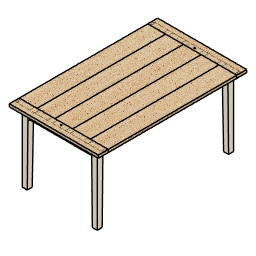
Farmhouse Table 2021 (Autodesk Fusion 360 design; units mm, degrees)
Autodesk Fusion 360 part; units mm, degrees
note: some values were not read from the file. Chosen so that the rebuilt part matches the saved one: which face or edge a step refers to; where a step ends. Set by a fixed rule: which sketch regions a step uses.
sketch "Sketch1" plane through (0, 0, 0) normal (1, 0, 0) x (0, 0, -1) in component "Breadboard"
  line L0 (0, 0) -> (-101.6, 0)
  line L1 (-101.6, 0) -> (-101.6, 28.575)
  line L2 (-101.6, 28.575) -> (0, 28.575)
  line L3 (0, 28.575) -> (0, 0)
  dimension "d1" = 28.575
  dimension "d2" = 101.6
  dimension "d215" = 0
  dimension "d216" = 0
  dimension "d217" = 0
  dimension "d218" = 0
  dimension "d275" = 0
  dimension "d276" = 0
  dimension "d277" = 0
  dimension "d278" = 0
  constraint horizontal L0
  constraint vertical L1
  constraint horizontal L2
  constraint vertical L3
  constraint coincident L0.start L3.end
  measures "d1" distance of L0.start L2.end
  measures "d2" distance of L0.start L0.end
extrude "Extrude1" add sketch "Sketch1" along normal blind 914.4 makes body 1 in component "Breadboard"
sketch "Sketch2" plane through (0, 0, 0) normal (0, 0, -1) x (-1, 0, 0) in component "Breadboard"
  line L0 (0, 0) -> (0, 28.575)
  line L1 (0, 28.575) -> (-914.4, 28.575)
  line L2 (-914.4, 28.575) -> (-914.4, 0)
  line L3 (-914.4, 0) -> (0, 0)
  line L4 (-901.7, 7.9375) -> (-12.7, 7.9375)
  line L5 (-12.7, 7.9375) -> (-12.7, 20.6375)
  line L6 (-12.7, 20.6375) -> (-901.7, 20.6375)
  line L7 (-901.7, 20.6375) -> (-901.7, 7.9375)
  line L8 (-901.7, 20.6375) -> (-901.7, 28.575) construction
  line L9 (-901.7, 7.9375) -> (-901.7, 0) construction
  line L10 (-12.7, 20.6375) -> (0, 20.6375) construction
  line L11 (-901.7, 20.6375) -> (-914.4, 20.6375) construction
  dimension "d7" = 12.7
  dimension "d11" = 12.7
  constraint horizontal L4
  constraint vertical L5
  constraint horizontal L6
  constraint vertical L7
  constraint coincident L1 L8.end
  constraint perpendicular L1 L8
  constraint coincident L3 L9.end
  constraint vertical L9
  constraint equal L8 L9
  constraint coincident L0 L10.end
  constraint coincident L2 L11.end
  constraint horizontal L11
  constraint horizontal L10
  constraint equal L10 L11
  measures "d7" vertical distance of L4.start L6.end
  measures "d11" distance of L2 L7
extrude "Extrude2" cut sketch "Sketch2" against normal blind 50.8 contours L4 L5 L6 L7 bodies 1 in component "Breadboard"
sketch "Sketch3" plane through (0, 28.575, 0) normal (0, 1, 0) x (-1, 0, 0) in component "Breadboard"
  line L0 (0, 0) -> (0, 101.6)
  line L1 (0, 101.6) -> (-914.4, 101.6)
  line L2 (-914.4, 101.6) -> (-914.4, 0)
  line L3 (-914.4, 0) -> (0, 0)
  line L4 (-457.2, 0) -> (-457.2, 25.4) construction
  circle A0 centre (-457.2, 25.4) radius 6.35
  dimension "d15" = 25.4
  dimension "d17" = 12.7
  constraint coincident L3 L4.start
  constraint perpendicular L3 L4
  constraint midpoint L3 L4.start
  constraint coincident L4.end A0.centre
  measures "d15" vertical distance of L4.start L4.end
  measures "d17" diameter of A0
extrude "Extrude3" cut sketch "Sketch3" against normal through all contours A0 bodies 1 in component "Breadboard"
sketch "Sketch1 (2)" plane through (0, 0, 0) normal (0, 0, 1) x (1, 0, 0) in component "Board"
  line L0 (0, 0) -> (182.88, 0)
  line L1 (182.88, 0) -> (182.88, 28.575)
  line L2 (182.88, 28.575) -> (0, 28.575)
  line L3 (0, 28.575) -> (0, 0)
  line L4 (0, 28.575) -> (914.4, 28.575)
  dimension "d22" = 182.88
  constraint horizontal L0
  constraint vertical L1
  constraint horizontal L2
  constraint vertical L3
  constraint coincident L1.end L4
  constraint coincident L0.start L3.end
  measures "d22" horizontal distance of L0.start L0.end
extrude "Extrude1'" add sketch "Sketch1 (2)" against normal blind 1320.8 separate body makes body 2 in component "Board"
ref_plane "WorkPlane1" through (91.44, 14.2875, -660.4) normal (0, 0, 1) x (1, 0, 0) in component "Board"
sketch "Sketch2 (2)" plane through (0, 0, 0) normal (0, 0, 1) x (1, 0, 0) in component "Board"
  line L0 (0, 0) -> (182.88, 0)
  line L1 (182.88, 0) -> (182.88, 28.575)
  line L2 (182.88, 28.575) -> (0, 28.575)
  line L3 (0, 28.575) -> (0, 0)
  line L4 (25.4, 7.9375) -> (157.48, 7.9375)
  line L5 (157.48, 7.9375) -> (157.48, 20.6375)
  line L6 (157.48, 20.6375) -> (25.4, 20.6375)
  line L7 (25.4, 20.6375) -> (25.4, 7.9375)
  line L8 (157.48, 7.9375) -> (157.48, 0) construction
  line L9 (157.48, 20.6375) -> (157.48, 28.575) construction
  line L10 (91.44, 28.575) -> (91.44, 0) construction
  dimension "d25" = 12.7
  dimension "d26" = 25.4
  constraint horizontal L4
  constraint vertical L5
  constraint horizontal L6
  constraint vertical L7
  constraint coincident L0 L8.end
  constraint coincident L2 L9.end
  constraint equal L8 L9
  constraint vertical L8
  constraint vertical L9
  constraint midpoint L2 L10.start
  constraint midpoint L0 L10.end
  constraint symmetric L5 L7 L10
  measures "d25" vertical distance of L4.start L6.end
  measures "d26" distance of L3 L7
extrude "Extrude2'" add sketch "Sketch2 (2)" along normal blind 50.8 contours L4 L5 L6 L7 bodies 2 in component "Board"
mirror "Mirror1" about plane through (91.44, 14.2875, -660.4) normal (0, 0, 1) of "Extrude2'" in component "Board"
sketch "Sketch1 (3)" plane through (0, 0, 0) normal (0, 0, 1) x (1, 0, 0) in component "Centerboard"
  line L0 (0, 0) -> (182.88, 0)
  line L1 (182.88, 0) -> (182.88, 28.575)
  line L2 (182.88, 28.575) -> (0, 28.575)
  line L3 (0, 28.575) -> (0, 0)
  line L4 (0, 28.575) -> (914.4, 28.575)
  dimension "d22_1" = 182.88
  constraint horizontal L0
  constraint vertical L1
  constraint horizontal L2
  constraint vertical L3
  constraint coincident L1.end L4
  constraint coincident L0.start L3.end
  measures "d22_1" horizontal distance of L0.start L0.end
extrude "Extrude1''" add sketch "Sketch1 (3)" against normal blind 1320.8 separate body makes body 3 in component "Centerboard"
ref_plane "WorkPlane1" through (91.44, 14.2875, -660.4) normal (0, 0, 1) x (1, 0, 0) in component "Centerboard"
sketch "Sketch2 (3)" plane through (0, 0, 0) normal (0, 0, 1) x (1, 0, 0) in component "Centerboard"
  line L0 (0, 0) -> (182.88, 0)
  line L1 (182.88, 0) -> (182.88, 28.575)
  line L2 (182.88, 28.575) -> (0, 28.575)
  line L3 (0, 28.575) -> (0, 0)
  line L4 (25.4, 7.9375) -> (157.48, 7.9375)
  line L5 (157.48, 7.9375) -> (157.48, 20.6375)
  line L6 (157.48, 20.6375) -> (25.4, 20.6375)
  line L7 (25.4, 20.6375) -> (25.4, 7.9375)
  line L8 (157.48, 7.9375) -> (157.48, 0) construction
  line L9 (157.48, 20.6375) -> (157.48, 28.575) construction
  line L10 (25.4, 20.6375) -> (25.4, 7.9375)
  line L11 (91.44, 28.575) -> (91.44, 0)
  dimension "d25_1" = 12.7
  dimension "d26_1" = 25.4
  constraint horizontal L4
  constraint vertical L5
  constraint horizontal L6
  constraint vertical L7
  constraint coincident L0 L8.end
  constraint coincident L2 L9.end
  constraint equal L8 L9
  constraint vertical L8
  constraint vertical L9
  measures "d25_1" vertical distance of L4.start L6.end
  measures "d26_1" distance of L3 L7
extrude "Extrude2''" add sketch "Sketch2 (3)" along normal blind 50.8 contours L4 L5 L6 L11 | L4 L6 L7 L10 L11 bodies 3 in component "Centerboard"
mirror "Mirror1'" about plane through (91.44, 14.2875, -660.4) normal (0, 0, 1) of "Extrude2''" in component "Centerboard"
sketch "Sketch3 (2)" plane through (0, 0, 0) normal (0, 1, 0) x (1, 0, 0) in component "Centerboard"
  circle A0 centre (91.44, -25.4) radius 6.35
  line L0 (25.4, -50.8) -> (157.48, -50.8)
  line L1 (91.44, -25.4) -> (91.44, -50.8) construction
  dimension "d30" = 12.7
  dimension "d31" = 25.4
  constraint coincident A0.centre L1.start
  constraint midpoint L0 L1.end
  constraint vertical L1
  measures "d30" diameter of A0
  measures "d31" vertical distance of A0.centre L1.end
extrude "Extrude3'" cut sketch "Sketch3 (2)" along normal up to surface (20.6375 mm away) bodies 3 in component "Centerboard"
mirror "Mirror2" about plane through (91.44, 14.2875, -660.4) normal (0, 0, 1) of "Extrude3'" in component "Centerboard"
sketch "Sketch1 (4)" plane through (0, 0, 0) normal (0, 1, 0) x (1, 0, 0) in component "Dowel"
  circle A0 centre (457.2, -25.4) radius 6.35
  circle A1 centre (457.2, -25.4) radius 6.35
  point P0 (463.55, -25.4)
  constraint coincident A0 P0
  constraint concentric A0 A1
extrude "Extrude1'''" add sketch "Sketch1 (4)" along normal blind 28.575 separate body makes body 4 in component "Dowel"
sketch "Sketch1 (5)" plane through (0, 0, 0) normal (0, 1, 0) x (1, 0, 0) in component "leg"
  line L0 (73.025, -28.575) -> (130.175, -28.575)
  line L1 (130.175, -28.575) -> (130.175, 28.575)
  line L2 (130.175, 28.575) -> (73.025, 28.575)
  line L3 (73.025, 28.575) -> (73.025, -28.575)
  line L4 (0, 0) -> (914.4, 0)
  line L5 (0, -101.6) -> (0, 0)
  line L6 (73.025, -28.575) -> (0, -28.575) construction
  line L7 (0, -101.6) -> (914.4, -101.6)
  line L8 (73.025, -28.575) -> (73.025, -101.6) construction
  dimension "d45" = 57.15
  dimension "d46" = 28.575
  constraint horizontal L0
  constraint vertical L1
  constraint horizontal L2
  constraint vertical L3
  constraint equal L0 L3
  constraint coincident L5 L6.end
  constraint coincident L7 L8.end
  constraint perpendicular L0 L8
  constraint horizontal L6
  constraint equal L6 L8
  measures "d45" horizontal distance of L0.start L0.end
  measures "d46" distance of L0 L4
extrude "Extrude1''''" add sketch "Sketch1 (5)" against normal blind 708.025 separate body makes body 5 in component "leg"
ref_plane "WorkPlane1" through (130.175, 0, -28.575) normal (0.707107, 0, 0.707107) x (0, 1, 0) in component "leg"
sketch "Sketch2 (4)" plane through (130.175, 0, 0) normal (1, 0, 0) x (0, 0, -1) in component "leg"
  line L0 (28.575, 0) -> (-28.575, 0)
  line L1 (-28.575, 0) -> (-28.575, -708.025)
  line L2 (-28.575, -708.025) -> (28.575, -708.025)
  line L3 (28.575, -708.025) -> (28.575, 0)
  line L4 (28.575, -89.154) -> (22.225, -708.025)
  dimension "d51" = 618.871
  dimension "d52" = 50.8
  constraint coincident L3 L4.start
  constraint coincident L2 L4.end
  measures "d51" distance of L2 L4.start
  measures "d52" distance of L1 L4.end
extrude "Extrude2'''" cut sketch "Sketch2 (4)" against normal up to surface (57.15 mm away) contours L2 L3 L4 bodies 5 in component "leg"
mirror "Mirror1''" about plane through (130.175, 0, -28.575) normal (0.707107, 0, 0.707107) of "Extrude2'''" in component "leg"
sketch "Sketch3 (3)" plane through (130.175, 0, 0) normal (1, 0, 0) x (0, 0, -1) in component "leg"
  line L0 (-28.575, -89.154) -> (28.575, -89.154)
  line L1 (28.575, -89.154) -> (28.575, 0)
  line L2 (28.575, 0) -> (-28.575, 0)
  line L3 (-28.575, 0) -> (-28.575, -89.154)
  line L4 (-6.35, 0) -> (6.35, 0)
  line L5 (6.35, 0) -> (6.35, -88.9)
  line L6 (6.35, -88.9) -> (-6.35, -88.9)
  line L7 (-6.35, -88.9) -> (-6.35, 0)
  dimension "d58" = 12.7
  dimension "d59" = 88.9
  constraint horizontal L4
  constraint vertical L5
  constraint horizontal L6
  constraint vertical L7
  constraint coincident L2 L4.start
  constraint midpoint L2 L4
  measures "d58" horizontal distance of L5.end L6.end
  measures "d59" vertical distance of L4.end L5.end
extrude "Extrude3''" cut sketch "Sketch3 (3)" against normal blind 25.4 contours L2 L4 L5 L6 L7 bodies 5 in component "leg"
mirror "Mirror2'" about plane through (130.175, 0, -28.575) normal (0.707107, 0, 0.707107) of "Extrude3''" in component "leg"
ref_plane "WorkPlane1" through (457.2, 14.2875, 50.8) normal (1, 0, 0) x (0, 0, -1)
ref_plane "WorkPlane2" through (457.2, 14.2875, -507.9861) normal (0, 0, 1) x (0, -1, 0)
mirror "MirrorComponent1" about plane through (0, 0, 0) normal (0, 0, 1) of bodies 5 makes body 6 in component "leg (1)"
mirror "MirrorComponent2" about plane through (0, 0, 0) normal (0, 0, 1) of bodies 5 makes body 7 in component "leg (2)"
mirror "MirrorComponent2'" about plane through (0, 0, 0) normal (0, 0, 1) of bodies 6 makes body 8 in component "leg (3)"
sketch "Sketch1 (6)" plane through (130.175, 0, 0) normal (1, 0, 0) x (0, 0, -1) in component "EndRail"
  line L0 (-6.35, -88.9) -> (-6.35, 0)
  line L1 (-6.35, 0) -> (-28.575, 0)
  line L2 (-28.575, 0) -> (-28.575, -89.154)
  line L3 (-28.575, -89.154) -> (28.575, -89.154)
  line L4 (28.575, -89.154) -> (28.575, 0)
  line L5 (28.575, 0) -> (6.35, 0)
  line L6 (6.35, 0) -> (6.35, -88.9)
  line L7 (-11.1125, 0) -> (11.1125, 0)
  line L8 (11.1125, 0) -> (11.1125, -88.9)
  line L9 (11.1125, -88.9) -> (-11.1125, -88.9)
  line L10 (-11.1125, -88.9) -> (-11.1125, 0)
  line L11 (6.35, -88.9) -> (-6.35, -88.9)
  line L12 (6.35, -88.9) -> (-6.35, -88.9)
  dimension "d63" = 22.225
  dimension "d211" = 0
  dimension "d212" = 0
  dimension "d213" = 0
  dimension "d214" = 0
  dimension "d271" = 0
  dimension "d272" = 0
  dimension "d273" = 0
  dimension "d274" = 0
  constraint horizontal L7
  constraint vertical L8
  constraint horizontal L9
  constraint vertical L10
  constraint midpoint L9 L11
  constraint collinear L1 L7
  measures "d63" horizontal distance of L8.end L9.end
extrude "Extrude1'''''" add sketch "Sketch1 (6)" along normal up to near side of body 6 placed x (-1, 0, 0) y (0, 1, 0) z (0, 0, -1) at (914.4, 0, 0) separate body contours L0 L1 L7 L9 L10 | L0 L6 L7 L9 L11 L12 | L5 L6 L7 L8 L9 makes body 9 in component "EndRail"
sketch "Sketch2 (5)" plane through (104.775, 0, 0) normal (1, 0, 0) x (0, 0, -1) in component "EndRail"
  line L0 (-6.35, -88.9) -> (3.175, -88.9)
  line L1 (3.175, 0) -> (-6.35, 0)
  line L2 (-6.35, 0) -> (-6.35, -88.9)
  line L3 (-6.35, 0) -> (3.175, 0)
  line L4 (3.175, 0) -> (3.175, -88.9)
  line L5 (3.175, -88.9) -> (-6.35, -88.9)
  line L6 (-6.35, -88.9) -> (-6.35, 0)
  line L7 (3.175, -88.9) -> (3.175, 0)
  constraint horizontal L3
  constraint vertical L4
  constraint horizontal L5
  constraint vertical L6
  constraint coincident L0.end L4.end
  constraint coincident L1.end L2.start
extrude "Extrude2''''" add sketch "Sketch2 (5)" along normal up to surface (25.4 mm away) bodies 9 in component "EndRail"
mirror "Mirror1'''" about plane through (457.2, 14.2875, 50.8) normal (1, 0, 0) of "Extrude2''''" in component "EndRail"
mirror "MirrorComponent3" about plane through (0, 0, 0) normal (0, 0, 1) of bodies 9 makes body 10 in component "EndRail (1)"
sketch "Sketch1 (7)" plane through (0, 0, -28.575) normal (0, 0, -1) x (-1, 0, 0) in component "SideRail"
  line L0 (-95.25, 0) -> (-95.25, -88.9)
  line L1 (-107.95, -88.9) -> (-107.95, 0)
  line L2 (-107.95, 0) -> (-130.175, 0)
  line L3 (-130.175, 0) -> (-130.175, -89.154)
  line L4 (-130.175, -89.154) -> (-73.025, -89.154)
  line L5 (-73.025, -89.154) -> (-73.025, 0)
  line L6 (-73.025, 0) -> (-95.25, 0)
  line L7 (-95.25, -88.9) -> (-107.95, -88.9)
sketch "Sketch2 (6)" plane through (0, 0, -28.575) normal (0, 0, -1) x (1, 0, 0) in component "SideRail"
  line L0 (112.7125, 0) -> (90.4875, 0)
  line L1 (90.4875, 0) -> (90.4875, 88.9)
  line L2 (90.4875, 88.9) -> (112.7125, 88.9)
  line L3 (112.7125, 88.9) -> (112.7125, 0)
  line L4 (107.95, 88.9) -> (95.25, 88.9)
  line L5 (73.025, 0) -> (95.25, 0)
  dimension "d69" = 22.225
  constraint horizontal L0
  constraint vertical L1
  constraint horizontal L2
  constraint vertical L3
  constraint midpoint L2 L4
  constraint collinear L0 L5
  measures "d69" horizontal distance of L1.end L2.end
sketch "Sketch3 (4)" plane through (0, 0, -3.175) normal (0, 0, -1) x (-1, 0, 0) in component "SideRail"
  line L0 (-95.25, -88.9) -> (-95.25, 0)
  line L1 (-95.25, 0) -> (-104.775, 0)
  line L2 (-104.775, 0) -> (-95.25, 0)
  line L3 (-95.25, 0) -> (-95.25, -88.9)
  line L4 (-95.25, -88.9) -> (-104.775, -88.9)
  line L5 (-104.775, -88.9) -> (-104.775, 0)
  line L6 (-104.775, 0) -> (-104.775, -88.9)
  line L7 (-104.775, -88.9) -> (-95.25, -88.9)
  constraint horizontal L2
  constraint vertical L3
  constraint horizontal L4
  constraint vertical L5
  constraint coincident L0.start L3.end
  constraint coincident L1.end L2.start
extrude "Extrude1''''''" add sketch "Sketch2 (6)" along normal blind 1285.875 separate body makes body 11 in component "SideRail"
extrude "Extrude2'''''" add 1 faces at (98.425, -29.6333, -3.175) along direction (0, 0, -1) up to surface (25.4 mm away) on bodies 5 bodies 11 in component "SideRail"
mirror "MirrorComponent4" about plane through (0, 0, 0) normal (0, 0, 1) of bodies 11 makes body 12 in component "SideRail(Mirror)"
mirror "MirrorComponent5" about plane through (0, 0, 0) normal (0, 0, 1) of bodies 4 makes body 13 in component "Dowel(Mirror)"
ref_plane "WorkPlane1" through (101.6, -44.45, -671.5125) normal (0, 0, -1) x (-1, 0, 0) in component "SideRail"
mirror "Mirror1''''" about plane through (101.6, -44.45, -671.5125) normal (0, 0, -1) of "Extrude2'''''" in component "SideRail"
component "Breadboard" placed x (1, 0, 0) y (0, 1, 0) z (0, 0, 1) at (12.5141, 179.7728, -151.6469)
component "Board" placed x (1, 0, 0) y (0, 1, 0) z (0, 0, 1) at (12.5141, 179.7728, -151.6469)
component "Centerboard" placed x (1, 0, 0) y (0, 1, 0) z (0, 0, 1) at (378.2741, 179.7728, -151.6469)
component "Board" placed x (1, 0, 0) y (0, 1, 0) z (0, 0, 1) at (195.3941, 179.7728, -151.6469)
component "Board" placed x (1, 0, 0) y (0, 1, 0) z (0, 0, 1) at (561.1541, 179.7728, -151.6469)
component "Board" placed x (1, 0, 0) y (0, 1, 0) z (0, 0, 1) at (744.0341, 179.7728, -151.6469)
component "Breadboard" placed x (1, 0, 0) y (0, -1, 0) z (0, 0, -1) at (12.5141, 208.3478, -1472.4469)
component "Dowel" placed x (0.972464, 0, -0.233054) y (0, 1, 0) z (0.233054, 0, 0.972464) at (19.184, 179.7728, -44.3953)
component "leg" placed x (1, 0, 0) y (0, 1, 0) z (0, 0, 1) at (12.5141, 179.7728, -138.9469)
component "EndRail" placed x (1, 0, 0) y (0, 1, 0) z (0, 0, 1) at (12.5141, 179.7728, -140.5344)
component "SideRail" placed x (1, 0, 0) y (0, 1, 0) z (0, 0, 1) at (12.5141, 179.7728, -138.9469)
component "Dowel(Mirror)" placed x (1, 0, 0) y (0, 1, 0) z (0, 0, 1) at (12.5141, 179.7728, -1472.4469)
component "leg (1)" placed x (-1, 0, 0) y (0, 1, 0) z (0, 0, -1) at (926.9141, 179.7728, -140.5344)
component "leg (2)" placed x (1, 0, 0) y (0, 1, 0) z (0, 0, 1) at (12.5141, 179.7728, -1483.5594)
component "leg (3)" placed x (-1, 0, 0) y (0, 1, 0) z (0, 0, -1) at (926.9141, 179.7728, -1483.5594)
component "EndRail (1)" placed x (1, 0, 0) y (0, 1, 0) z (0, 0, 1) at (12.5141, 179.7728, -1483.5594)
component "SideRail(Mirror)" placed x (-1, 0, 0) y (0, 1, 0) z (0, 0, -1) at (926.9141, 179.7728, -140.5344)
equation "d1 = top_thickness"
equation "d2 = breadboard_width"
equation "top_thickness = 1.125 in"
equation "d4 = width"
equation "d7 = tenon_thickness"
equation "tenon_thickness = 0.5 in"
equation "d11 = tenon_thickness"
equation "d12 = -tenon_length"
equation "tenon_length = 2 in"
equation "d15 = tenon_length / 2"
equation "dowel_thickness = 0.5 in"
equation "d17 = dowel_thickness"
equation "width = 36 in"
equation "length = 60 in"
equation "breadboard_width = 4 in"
equation "d22 = width / 5"
equation "d23 = -length + 2 * breadboard_width"
equation "d25 = tenon_thickness"
equation "d26 = tenon_thickness * 2"
equation "d27 = tenon_length"
equation "d22_1 = width / 5"
equation "d23_1 = -length + 2 * breadboard_width"
equation "d25_1 = tenon_thickness"
equation "d26_1 = tenon_thickness * 2"
equation "d27_1 = tenon_length"
equation "d30 = dowel_thickness"
equation "d31 = tenon_length / 2"
equation "d36 = top_thickness"
equation "rail_thickness = 0.875 in"
equation "rail_height = 3.5 in"
equation "leg_thickness = 2.25 in"
equation "leg_height = height - top_thickness"
equation "d45 = leg_thickness"
equation "d46 = leg_thickness / 2"
equation "d47 = -leg_height"
equation "leg_taperthickness = 2 in"
equation "leg_taperheight = leg_height - rail_height - 0.01 in"
equation "d51 = leg_taperheight"
equation "d52 = leg_taperthickness"
equation "d58 = tenon_thickness"
equation "d59 = rail_height"
equation "d60 = -tenon_length / 2"
equation "d63 = rail_thickness"
equation "d69 = rail_thickness"
equation "overhang = 3 in"
equation "d327 = length - 2 * breadboard_width - leg_thickness + rail_thickness"
equation "height = 29 in"
